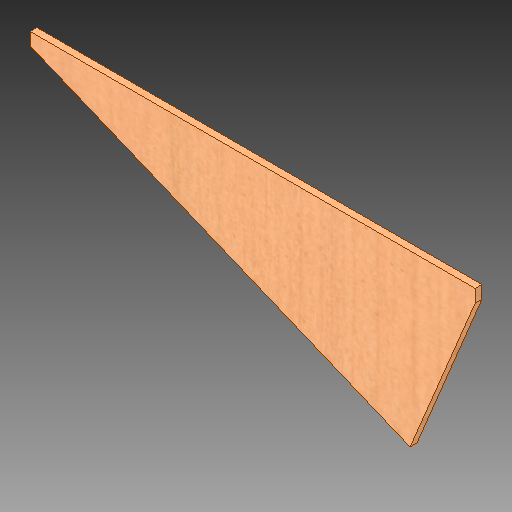
# Autodesk Inventor part: ref3
Saved by Autodesk Inventor 2019 (Build 230136000, 136)
## iProperties
Created: 2019-01-08
Part Number: ref3
Material: Wood (Cherry)
Document SubType Name: Modeling
Designer: gaincarlo
Density: 0.63 g/cm^3
Appearance: Cherry - Natural Low Gloss
Author: gaincarlo
Autodesk Inventor part; units mm, degrees
ref_plane "YZ Plane" through (0, 0, 0) normal (1, 0, 0) x (0, 1, 0)
ref_plane "XZ Plane" through (0, 0, 0) normal (0, 1, 0) x (-1, 0, 0)
ref_plane "Work Plane1" through (0, 0, 0) normal (0, 0, 1) x (1, 0, 0)
sketch "Sketch1" plane through (0, 0, 0) normal (0, 0, 1) x (1, 0, 0)
  line L0 (11.4028, 292.4518) -> (-26.8656, 200.0638) projected
  line L1 (-250.5009, 292.6966) -> (303.8268, 63.0866) projected
  line L2 (300, 300) -> (-300, 300) projected
  line L3 (11.4028, 292.4518) -> (11.4028, 300)
  line L4 (-250.5009, 292.6966) -> (-250.5009, 300)
  point P0 (0, 0)
  constraints: 4 end point, 2 perpendicular, 2 point on line, 1 vertical
extrude "Extrusion1" add sketch "Sketch1" along normal blind 4
body "Solid1"
